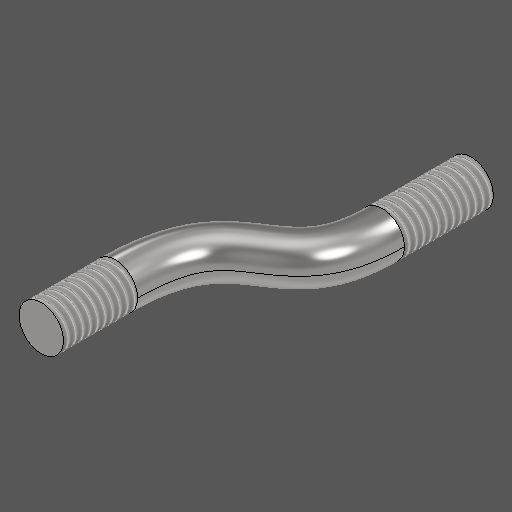
# Autodesk Inventor part: m3-pin-bent-6mm
Saved by Autodesk Inventor 2025 (Build 290162000, 162)
## iProperties
Created: 2024-05-16
Part Number: m3-pin-bent-6mm
Material: Stainless Steel
Document SubType Name: Modeling
Designer: kuzmin
Density: 8 g/cm^3
Appearance: Semi-Polished
Author: kuzmin
Autodesk Inventor part; units mm, degrees
ref_plane "YZ Plane" through (0, 0, 0) normal (1, 0, 0) x (0, 1, 0)
ref_plane "XZ Plane" through (0, 0, 0) normal (0, 1, 0) x (-1, 0, 0)
ref_plane "XY Plane" through (0, 0, 0) normal (0, 0, 1) x (1, 0, 0)
sketch "Sketch1" plane through (0, 0, 0) normal (0, 0, 1) x (1, 0, 0)
  circle A0 centre (0, 0) radius 1.5
  dimension "d0" = 3
  constraints: 1 centre point, 1 coincident
  measures "d0" diameter of A0
sketch "Sketch2" plane through (0, 0, 0) normal (0, 1, 0) x (-1, 0, 0)
  line L0 (0, 0) -> (0, 6)
  line L1 (6, 23) -> (6, 18)
  line L2 (6, 18) -> (6, 9.2623) construction
  spline S0 degree 3 poles (6, 18) (6, 9.2623) (0, 13.2145) (0, 6) knots 1 1 1 1 2 2 2 2
  line L3 (0, 13.2145) -> (0, 6) construction
  line L4 (6, 9.2623) -> (0, 13.2145) construction
  dimension "d1" = 6
  dimension "d3" = 23
  dimension "d4" = 6
  dimension "d11" = 5
  constraints: 4 end point, 4 vertical, 3 other
  measures "d1" distance between parallel lines of L0 L1
  measures "d3" vertical distance of L0.start L1.start
  measures "d4" distance of L0.start L0.end
  measures "d11" distance of L1.start L1.end
sweep "Sweep1" add profiles "Sketch1" path "Sketch2"
thread "Thread1"
thread "Thread2"
body "Solid1"
